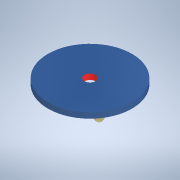
# Autodesk Inventor part: pll-base
Saved by Autodesk Inventor 2020 (Build 240168000, 168)
## iProperties
Created: 2020-12-11
Part Number: pll-base
Material: Generic
Document SubType Name: Modeling
Designer: Vikki
Density: 1 g/cm^3
Appearance: Default
Author: Vikki
Autodesk Inventor part; units mm, degrees
ref_plane "YZ Plane" through (0, 0, 0) normal (1, 0, 0) x (0, 1, 0)
ref_plane "XZ Plane" through (0, 0, 0) normal (0, 1, 0) x (-1, 0, 0)
ref_plane "XY Plane" through (0, 0, 0) normal (0, 0, 1) x (1, 0, 0)
sketch "Sketch1" plane through (0, 0, 0) normal (0, 1, 0) x (-1, 0, 0)
  circle A0 centre (0, 0) radius 63.5
  dimension "d0" = 127
  constraints: 1 centre point, 1 coincident
  measures "d0" diameter of A0
extrude "Extrusion1" add sketch "Sketch1" along normal blind 10
sketch "Sketch2" plane through (0, 0, 0) normal (0, -1, 0) x (1, 0, 0)
  circle A0 centre (0, -44.45) radius 5
  line L0 (0, 0) -> (0, -44.45)
  dimension "d3" = 44.45
  dimension "d4" = 10
  constraints: 2 end point, 1 centre point, 1 vertical
  measures "d3" distance of L0.start L0.end
  measures "d4" diameter of A0
extrude "Extrusion2" add sketch "Sketch2" along normal blind 20
sketch "Sketch3" plane through (0, -20, -44.45) normal (0, -1, 0) x (1, 0, 0)
  circle A0 centre (0, 0) radius 5 projected
  arc A1 (0, -7.5) -> (0, 7.5) centre (0, 0) ccw
  line L0 (0, 0) -> (0, -7.5)
  line L1 (0, 0) -> (0, 7.5)
  point P0 (0, 44.45)
  dimension "d7" = 7.5
  constraints: 4 end point, 2 point on circle, 1 centre point, 1 coincident, 1 point on line
  measures "d7" radius of A1
revolve "Revolution1" add sketch "Sketch3" angle 360 about axis through (0, -20, -44.45) along (0, 0, -1) picked at (1.094, -3.1265) contours A0 L0 L1 | A0 L1 A1 L0
pattern_circular "Circular Pattern1" count 3 over 360 about axis through (0, -10, 0) along (0, 1, 0) of "Extrusion2", "Revolution1"
sketch "Sketch4" plane through (0, 10, 0) normal (0, 1, 0) x (1, 0, 0)
  circle A0 centre (0, 0) radius 10
  dimension "d12" = 20
  constraints: 1 centre point, 1 coincident
  measures "d12" diameter of A0
extrude "Extrusion3" cut sketch "Sketch4" against normal up to surface (10 mm away)
body "Solid1"
